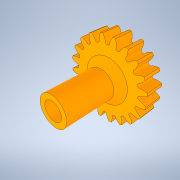
# Autodesk Inventor part: Шестерня мотора
Saved by Autodesk Inventor 2021.1 (Build 251245010, 245A)
## iProperties
Created: 2026-05-06
Part Number: Шестерня мотора
Material: Generic
Document SubType Name: Modeling
Designer: Андрей Тарасов
Density: 1 g/cm^3
Appearance: Default
Author: Андрей Тарасов
Autodesk Inventor part; units mm, degrees
ref_plane "YZ Plane" through (0, 0, 0) normal (1, 0, 0) x (0, 1, 0)
ref_plane "XZ Plane" through (0, 0, 0) normal (0, 1, 0) x (-1, 0, 0)
ref_plane "XY Plane" through (0, 0, 0) normal (0, 0, 1) x (1, 0, 0)
sketch "Sketch1" plane through (0, 0, 0) normal (0, 0, 1) x (1, 0, 0)
  spline S0 degree 3 poles (-1.3768, 10.9135) (-1.3416, 10.8686) (-1.2712, 10.7789) (-1.1713, 10.64) (-1.0757, 10.4981) (-0.9853, 10.3528) (-0.9005, 10.2042) (-0.8221, 10.0521) (-0.7507, 9.8965) (-0.6878, 9.7374) (-0.6438, 9.6016) (-0.616, 9.4911) (-0.5991, 9.407) (-0.5929, 9.3216) (-0.5783, 9.2373) (-0.5604, 9.1536) (-0.5337, 9.0722) (-0.5001, 8.9934) (-0.4629, 8.9323) (-0.4286, 8.8868) (-0.3992, 8.8556) (-0.3672, 8.8271) (-0.3323, 8.8024) (-0.2946, 8.782) (-0.2551, 8.7654) (-0.2137, 8.7543) (-0.1284, 8.7448) (0, 8.7541) (0.1284, 8.7448) (0.2137, 8.7543) (0.2551, 8.7654) (0.2946, 8.782) (0.3323, 8.8024) (0.3672, 8.8271) (0.3992, 8.8556) (0.4286, 8.8868) (0.4629, 8.9323) (0.5001, 8.9934) (0.5337, 9.0722) (0.5604, 9.1536) (0.5783, 9.2373) (0.5929, 9.3216) (0.5991, 9.407) (0.616, 9.4911) (0.6438, 9.6016) (0.6878, 9.7374) (0.7507, 9.8965) (0.8221, 10.0521) (0.9005, 10.2042) (0.9853, 10.3528) (1.0757, 10.4981) (1.1713, 10.64) (1.2712, 10.7789) (1.3416, 10.8686) (1.3768, 10.9135) knots 0 0 0 0 0.017107 0.034214 0.051321 0.068427 0.085534 0.10264 0.119746 0.136852 0.153955 0.162508 0.17106 0.179613 0.188166 0.196719 0.20527 0.213818 0.222364 0.22664 0.230917 0.235193 0.239468 0.24374 0.248014 0.252292 0.256565 0.273669 0.290774 0.295047 0.299325 0.303599 0.307871 0.312146 0.316422 0.320699 0.324975 0.333521 0.342069 0.35062 0.359172 0.367726 0.376279 0.384831 0.393384 0.410487 0.427593 0.444699 0.461805 0.478912 0.496018 0.513125 0.530232 0.547339 0.547339 0.547339 0.547339
  circle A0 centre (0, 0) radius 8.75 construction
  circle A1 centre (0, 0) radius 9.3969 construction
  circle A2 centre (0, 0) radius 10 construction
  circle A3 centre (0, 0) radius 11
  spline S1 degree 3 poles (-4.6819, 9.9539) (-4.6345, 9.9221) (-4.5399, 9.8585) (-4.4019, 9.7573) (-4.2671, 9.6518) (-4.1363, 9.5416) (-4.0097, 9.4264) (-3.8881, 9.3061) (-3.7722, 9.1802) (-3.6632, 9.0483) (-3.5794, 8.9328) (-3.5187, 8.8362) (-3.4768, 8.7615) (-3.4444, 8.6822) (-3.4045, 8.6065) (-3.3616, 8.5324) (-3.311, 8.4633) (-3.2548, 8.3987) (-3.2005, 8.3521) (-3.1538, 8.3194) (-3.1162, 8.2988) (-3.077, 8.2816) (-3.0361, 8.2689) (-2.994, 8.2612) (-2.9513, 8.2575) (-2.9084, 8.2598) (-2.8244, 8.2771) (-2.7052, 8.3257) (-2.5801, 8.3565) (-2.502, 8.3918) (-2.466, 8.4152) (-2.4336, 8.4432) (-2.4041, 8.4742) (-2.3785, 8.5086) (-2.3568, 8.5455) (-2.3385, 8.5843) (-2.32, 8.6382) (-2.3034, 8.7078) (-2.2959, 8.7931) (-2.2957, 8.8787) (-2.3045, 8.9639) (-2.3166, 9.0486) (-2.3371, 9.1318) (-2.3471, 9.2169) (-2.3548, 9.3306) (-2.3549, 9.4734) (-2.3442, 9.6442) (-2.3244, 9.8141) (-2.2968, 9.983) (-2.2621, 10.1506) (-2.221, 10.3167) (-2.1739, 10.4812) (-2.1218, 10.6441) (-2.0826, 10.7513) (-2.063, 10.8048) knots 0 0 0 0 0.017107 0.034214 0.051321 0.068427 0.085534 0.10264 0.119746 0.136852 0.153955 0.162508 0.17106 0.179613 0.188166 0.196719 0.20527 0.213818 0.222364 0.22664 0.230917 0.235193 0.239468 0.24374 0.248014 0.252292 0.256565 0.273669 0.290774 0.295047 0.299325 0.303599 0.307871 0.312146 0.316422 0.320699 0.324975 0.333521 0.342069 0.35062 0.359172 0.367726 0.376279 0.384831 0.393384 0.410487 0.427593 0.444699 0.461805 0.478912 0.496018 0.513125 0.530232 0.547339 0.547339 0.547339 0.547339
  spline S2 degree 3 poles (-7.5287, 8.0199) (-7.4738, 8.0043) (-7.3641, 7.9731) (-7.2016, 7.9194) (-7.0409, 7.8608) (-6.8824, 7.7964) (-6.7264, 7.726) (-6.5735, 7.6491) (-6.4244, 7.5652) (-6.28, 7.4734) (-6.1646, 7.3895) (-6.077, 7.3164) (-6.014, 7.2583) (-5.9588, 7.1928) (-5.8974, 7.1332) (-5.8337, 7.076) (-5.7643, 7.0259) (-5.6908, 6.9818) (-5.6248, 6.9543) (-5.5703, 6.9376) (-5.5282, 6.9296) (-5.4855, 6.9254) (-5.4427, 6.926) (-5.4003, 6.9316) (-5.3585, 6.9414) (-5.3185, 6.9568) (-5.244, 6.9992) (-5.1456, 7.0823) (-5.0362, 7.1502) (-4.9728, 7.2079) (-4.9458, 7.2413) (-4.9236, 7.2779) (-4.9051, 7.3166) (-4.8913, 7.3571) (-4.8822, 7.399) (-4.8768, 7.4415) (-4.8758, 7.4985) (-4.8815, 7.5698) (-4.9008, 7.6533) (-4.927, 7.7348) (-4.9617, 7.813) (-4.9994, 7.8899) (-5.0446, 7.9626) (-5.0804, 8.0405) (-5.1228, 8.1463) (-5.167, 8.282) (-5.2097, 8.4477) (-5.2434, 8.6155) (-5.2693, 8.7847) (-5.2881, 8.9547) (-5.3003, 9.1254) (-5.3064, 9.2964) (-5.3072, 9.4675) (-5.303, 9.5815) (-5.3009, 9.6385) knots 0 0 0 0 0.017107 0.034214 0.051321 0.068427 0.085534 0.10264 0.119746 0.136852 0.153955 0.162508 0.17106 0.179613 0.188166 0.196719 0.20527 0.213818 0.222364 0.22664 0.230917 0.235193 0.239468 0.24374 0.248014 0.252292 0.256565 0.273669 0.290774 0.295047 0.299325 0.303599 0.307871 0.312146 0.316422 0.320699 0.324975 0.333521 0.342069 0.35062 0.359172 0.367726 0.376279 0.384831 0.393384 0.410487 0.427593 0.444699 0.461805 0.478912 0.496018 0.513125 0.530232 0.547339 0.547339 0.547339 0.547339
  spline S3 degree 3 poles (-9.6385, 5.3009) (-9.5815, 5.303) (-9.4675, 5.3072) (-9.2964, 5.3064) (-9.1254, 5.3003) (-8.9547, 5.2881) (-8.7847, 5.2693) (-8.6155, 5.2434) (-8.4477, 5.2097) (-8.282, 5.167) (-8.1463, 5.1228) (-8.0405, 5.0804) (-7.9626, 5.0446) (-7.8899, 4.9994) (-7.813, 4.9617) (-7.7348, 4.927) (-7.6533, 4.9008) (-7.5698, 4.8815) (-7.4985, 4.8758) (-7.4415, 4.8768) (-7.399, 4.8822) (-7.3571, 4.8913) (-7.3166, 4.9051) (-7.2779, 4.9236) (-7.2413, 4.9458) (-7.2079, 4.9728) (-7.1502, 5.0362) (-7.0823, 5.1456) (-6.9992, 5.244) (-6.9568, 5.3185) (-6.9414, 5.3585) (-6.9316, 5.4003) (-6.926, 5.4427) (-6.9254, 5.4855) (-6.9296, 5.5282) (-6.9376, 5.5703) (-6.9543, 5.6248) (-6.9818, 5.6908) (-7.0259, 5.7643) (-7.076, 5.8337) (-7.1332, 5.8974) (-7.1928, 5.9588) (-7.2583, 6.014) (-7.3164, 6.077) (-7.3895, 6.1646) (-7.4734, 6.28) (-7.5652, 6.4244) (-7.6491, 6.5735) (-7.726, 6.7264) (-7.7964, 6.8824) (-7.8608, 7.0409) (-7.9194, 7.2016) (-7.9731, 7.3641) (-8.0043, 7.4738) (-8.0199, 7.5287) knots 0 0 0 0 0.017107 0.034214 0.051321 0.068427 0.085534 0.10264 0.119746 0.136852 0.153955 0.162508 0.17106 0.179613 0.188166 0.196719 0.20527 0.213818 0.222364 0.22664 0.230917 0.235193 0.239468 0.24374 0.248014 0.252292 0.256565 0.273669 0.290774 0.295047 0.299325 0.303599 0.307871 0.312146 0.316422 0.320699 0.324975 0.333521 0.342069 0.35062 0.359172 0.367726 0.376279 0.384831 0.393384 0.410487 0.427593 0.444699 0.461805 0.478912 0.496018 0.513125 0.530232 0.547339 0.547339 0.547339 0.547339
  spline S4 degree 3 poles (-10.8048, 2.063) (-10.7513, 2.0826) (-10.6441, 2.1218) (-10.4812, 2.1739) (-10.3167, 2.221) (-10.1506, 2.2621) (-9.983, 2.2968) (-9.8141, 2.3244) (-9.6442, 2.3442) (-9.4734, 2.3549) (-9.3306, 2.3548) (-9.2169, 2.3471) (-9.1318, 2.3371) (-9.0486, 2.3166) (-8.9639, 2.3045) (-8.8787, 2.2957) (-8.7931, 2.2959) (-8.7078, 2.3034) (-8.6382, 2.32) (-8.5843, 2.3385) (-8.5455, 2.3568) (-8.5086, 2.3785) (-8.4742, 2.4041) (-8.4432, 2.4336) (-8.4152, 2.466) (-8.3918, 2.502) (-8.3565, 2.5801) (-8.3257, 2.7052) (-8.2771, 2.8244) (-8.2598, 2.9084) (-8.2575, 2.9513) (-8.2612, 2.994) (-8.2689, 3.0361) (-8.2816, 3.077) (-8.2988, 3.1162) (-8.3194, 3.1538) (-8.3521, 3.2005) (-8.3987, 3.2548) (-8.4633, 3.311) (-8.5324, 3.3616) (-8.6065, 3.4045) (-8.6822, 3.4444) (-8.7615, 3.4768) (-8.8362, 3.5187) (-8.9328, 3.5794) (-9.0483, 3.6632) (-9.1802, 3.7722) (-9.3061, 3.8881) (-9.4264, 4.0097) (-9.5416, 4.1363) (-9.6518, 4.2671) (-9.7573, 4.4019) (-9.8585, 4.5399) (-9.9221, 4.6345) (-9.9539, 4.6819) knots 0 0 0 0 0.017107 0.034214 0.051321 0.068427 0.085534 0.10264 0.119746 0.136852 0.153955 0.162508 0.17106 0.179613 0.188166 0.196719 0.20527 0.213818 0.222364 0.22664 0.230917 0.235193 0.239468 0.24374 0.248014 0.252292 0.256565 0.273669 0.290774 0.295047 0.299325 0.303599 0.307871 0.312146 0.316422 0.320699 0.324975 0.333521 0.342069 0.35062 0.359172 0.367726 0.376279 0.384831 0.393384 0.410487 0.427593 0.444699 0.461805 0.478912 0.496018 0.513125 0.530232 0.547339 0.547339 0.547339 0.547339
  spline S5 degree 3 poles (-10.9135, -1.3768) (-10.8686, -1.3416) (-10.7789, -1.2712) (-10.64, -1.1713) (-10.4981, -1.0757) (-10.3528, -0.9853) (-10.2042, -0.9005) (-10.0521, -0.8221) (-9.8965, -0.7507) (-9.7374, -0.6878) (-9.6016, -0.6438) (-9.4911, -0.616) (-9.407, -0.5991) (-9.3216, -0.5929) (-9.2373, -0.5783) (-9.1536, -0.5604) (-9.0722, -0.5337) (-8.9934, -0.5001) (-8.9323, -0.4629) (-8.8868, -0.4286) (-8.8556, -0.3992) (-8.8271, -0.3672) (-8.8024, -0.3323) (-8.782, -0.2946) (-8.7654, -0.2551) (-8.7543, -0.2137) (-8.7448, -0.1284) (-8.7541, 0) (-8.7448, 0.1284) (-8.7543, 0.2137) (-8.7654, 0.2551) (-8.782, 0.2946) (-8.8024, 0.3323) (-8.8271, 0.3672) (-8.8556, 0.3992) (-8.8868, 0.4286) (-8.9323, 0.4629) (-8.9934, 0.5001) (-9.0722, 0.5337) (-9.1536, 0.5604) (-9.2373, 0.5783) (-9.3216, 0.5929) (-9.407, 0.5991) (-9.4911, 0.616) (-9.6016, 0.6438) (-9.7374, 0.6878) (-9.8965, 0.7507) (-10.0521, 0.8221) (-10.2042, 0.9005) (-10.3528, 0.9853) (-10.4981, 1.0757) (-10.64, 1.1713) (-10.7789, 1.2712) (-10.8686, 1.3416) (-10.9135, 1.3768) knots 0 0 0 0 0.017107 0.034214 0.051321 0.068427 0.085534 0.10264 0.119746 0.136852 0.153955 0.162508 0.17106 0.179613 0.188166 0.196719 0.20527 0.213818 0.222364 0.22664 0.230917 0.235193 0.239468 0.24374 0.248014 0.252292 0.256565 0.273669 0.290774 0.295047 0.299325 0.303599 0.307871 0.312146 0.316422 0.320699 0.324975 0.333521 0.342069 0.35062 0.359172 0.367726 0.376279 0.384831 0.393384 0.410487 0.427593 0.444699 0.461805 0.478912 0.496018 0.513125 0.530232 0.547339 0.547339 0.547339 0.547339
  spline S6 degree 3 poles (-9.9539, -4.6819) (-9.9221, -4.6345) (-9.8585, -4.5399) (-9.7573, -4.4019) (-9.6518, -4.2671) (-9.5416, -4.1363) (-9.4264, -4.0097) (-9.3061, -3.8881) (-9.1802, -3.7722) (-9.0483, -3.6632) (-8.9328, -3.5794) (-8.8362, -3.5187) (-8.7615, -3.4768) (-8.6822, -3.4444) (-8.6065, -3.4045) (-8.5324, -3.3616) (-8.4633, -3.311) (-8.3987, -3.2548) (-8.3521, -3.2005) (-8.3194, -3.1538) (-8.2988, -3.1162) (-8.2816, -3.077) (-8.2689, -3.0361) (-8.2612, -2.994) (-8.2575, -2.9513) (-8.2598, -2.9084) (-8.2771, -2.8244) (-8.3257, -2.7052) (-8.3565, -2.5801) (-8.3918, -2.502) (-8.4152, -2.466) (-8.4432, -2.4336) (-8.4742, -2.4041) (-8.5086, -2.3785) (-8.5455, -2.3568) (-8.5843, -2.3385) (-8.6382, -2.32) (-8.7078, -2.3034) (-8.7931, -2.2959) (-8.8787, -2.2957) (-8.9639, -2.3045) (-9.0486, -2.3166) (-9.1318, -2.3371) (-9.2169, -2.3471) (-9.3306, -2.3548) (-9.4734, -2.3549) (-9.6442, -2.3442) (-9.8141, -2.3244) (-9.983, -2.2968) (-10.1506, -2.2621) (-10.3167, -2.221) (-10.4812, -2.1739) (-10.6441, -2.1218) (-10.7513, -2.0826) (-10.8048, -2.063) knots 0 0 0 0 0.017107 0.034214 0.051321 0.068427 0.085534 0.10264 0.119746 0.136852 0.153955 0.162508 0.17106 0.179613 0.188166 0.196719 0.20527 0.213818 0.222364 0.22664 0.230917 0.235193 0.239468 0.24374 0.248014 0.252292 0.256565 0.273669 0.290774 0.295047 0.299325 0.303599 0.307871 0.312146 0.316422 0.320699 0.324975 0.333521 0.342069 0.35062 0.359172 0.367726 0.376279 0.384831 0.393384 0.410487 0.427593 0.444699 0.461805 0.478912 0.496018 0.513125 0.530232 0.547339 0.547339 0.547339 0.547339
  spline S7 degree 3 poles (-8.0199, -7.5287) (-8.0043, -7.4738) (-7.9731, -7.3641) (-7.9194, -7.2016) (-7.8608, -7.0409) (-7.7964, -6.8824) (-7.726, -6.7264) (-7.6491, -6.5735) (-7.5652, -6.4244) (-7.4734, -6.28) (-7.3895, -6.1646) (-7.3164, -6.077) (-7.2583, -6.014) (-7.1928, -5.9588) (-7.1332, -5.8974) (-7.076, -5.8337) (-7.0259, -5.7643) (-6.9818, -5.6908) (-6.9543, -5.6248) (-6.9376, -5.5703) (-6.9296, -5.5282) (-6.9254, -5.4855) (-6.926, -5.4427) (-6.9316, -5.4003) (-6.9414, -5.3585) (-6.9568, -5.3185) (-6.9992, -5.244) (-7.0823, -5.1456) (-7.1502, -5.0362) (-7.2079, -4.9728) (-7.2413, -4.9458) (-7.2779, -4.9236) (-7.3166, -4.9051) (-7.3571, -4.8913) (-7.399, -4.8822) (-7.4415, -4.8768) (-7.4985, -4.8758) (-7.5698, -4.8815) (-7.6533, -4.9008) (-7.7348, -4.927) (-7.813, -4.9617) (-7.8899, -4.9994) (-7.9626, -5.0446) (-8.0405, -5.0804) (-8.1463, -5.1228) (-8.282, -5.167) (-8.4477, -5.2097) (-8.6155, -5.2434) (-8.7847, -5.2693) (-8.9547, -5.2881) (-9.1254, -5.3003) (-9.2964, -5.3064) (-9.4675, -5.3072) (-9.5815, -5.303) (-9.6385, -5.3009) knots 0 0 0 0 0.017107 0.034214 0.051321 0.068427 0.085534 0.10264 0.119746 0.136852 0.153955 0.162508 0.17106 0.179613 0.188166 0.196719 0.20527 0.213818 0.222364 0.22664 0.230917 0.235193 0.239468 0.24374 0.248014 0.252292 0.256565 0.273669 0.290774 0.295047 0.299325 0.303599 0.307871 0.312146 0.316422 0.320699 0.324975 0.333521 0.342069 0.35062 0.359172 0.367726 0.376279 0.384831 0.393384 0.410487 0.427593 0.444699 0.461805 0.478912 0.496018 0.513125 0.530232 0.547339 0.547339 0.547339 0.547339
  spline S8 degree 3 poles (-5.3009, -9.6385) (-5.303, -9.5815) (-5.3072, -9.4675) (-5.3064, -9.2964) (-5.3003, -9.1254) (-5.2881, -8.9547) (-5.2693, -8.7847) (-5.2434, -8.6155) (-5.2097, -8.4477) (-5.167, -8.282) (-5.1228, -8.1463) (-5.0804, -8.0405) (-5.0446, -7.9626) (-4.9994, -7.8899) (-4.9617, -7.813) (-4.927, -7.7348) (-4.9008, -7.6533) (-4.8815, -7.5698) (-4.8758, -7.4985) (-4.8768, -7.4415) (-4.8822, -7.399) (-4.8913, -7.3571) (-4.9051, -7.3166) (-4.9236, -7.2779) (-4.9458, -7.2413) (-4.9728, -7.2079) (-5.0362, -7.1502) (-5.1456, -7.0823) (-5.244, -6.9992) (-5.3185, -6.9568) (-5.3585, -6.9414) (-5.4003, -6.9316) (-5.4427, -6.926) (-5.4855, -6.9254) (-5.5282, -6.9296) (-5.5703, -6.9376) (-5.6248, -6.9543) (-5.6908, -6.9818) (-5.7643, -7.0259) (-5.8337, -7.076) (-5.8974, -7.1332) (-5.9588, -7.1928) (-6.014, -7.2583) (-6.077, -7.3164) (-6.1646, -7.3895) (-6.28, -7.4734) (-6.4244, -7.5652) (-6.5735, -7.6491) (-6.7264, -7.726) (-6.8824, -7.7964) (-7.0409, -7.8608) (-7.2016, -7.9194) (-7.3641, -7.9731) (-7.4738, -8.0043) (-7.5287, -8.0199) knots 0 0 0 0 0.017107 0.034214 0.051321 0.068427 0.085534 0.10264 0.119746 0.136852 0.153955 0.162508 0.17106 0.179613 0.188166 0.196719 0.20527 0.213818 0.222364 0.22664 0.230917 0.235193 0.239468 0.24374 0.248014 0.252292 0.256565 0.273669 0.290774 0.295047 0.299325 0.303599 0.307871 0.312146 0.316422 0.320699 0.324975 0.333521 0.342069 0.35062 0.359172 0.367726 0.376279 0.384831 0.393384 0.410487 0.427593 0.444699 0.461805 0.478912 0.496018 0.513125 0.530232 0.547339 0.547339 0.547339 0.547339
  spline S9 degree 3 poles (-2.063, -10.8048) (-2.0826, -10.7513) (-2.1218, -10.6441) (-2.1739, -10.4812) (-2.221, -10.3167) (-2.2621, -10.1506) (-2.2968, -9.983) (-2.3244, -9.8141) (-2.3442, -9.6442) (-2.3549, -9.4734) (-2.3548, -9.3306) (-2.3471, -9.2169) (-2.3371, -9.1318) (-2.3166, -9.0486) (-2.3045, -8.9639) (-2.2957, -8.8787) (-2.2959, -8.7931) (-2.3034, -8.7078) (-2.32, -8.6382) (-2.3385, -8.5843) (-2.3568, -8.5455) (-2.3785, -8.5086) (-2.4041, -8.4742) (-2.4336, -8.4432) (-2.466, -8.4152) (-2.502, -8.3918) (-2.5801, -8.3565) (-2.7052, -8.3257) (-2.8244, -8.2771) (-2.9084, -8.2598) (-2.9513, -8.2575) (-2.994, -8.2612) (-3.0361, -8.2689) (-3.077, -8.2816) (-3.1162, -8.2988) (-3.1538, -8.3194) (-3.2005, -8.3521) (-3.2548, -8.3987) (-3.311, -8.4633) (-3.3616, -8.5324) (-3.4045, -8.6065) (-3.4444, -8.6822) (-3.4768, -8.7615) (-3.5187, -8.8362) (-3.5794, -8.9328) (-3.6632, -9.0483) (-3.7722, -9.1802) (-3.8881, -9.3061) (-4.0097, -9.4264) (-4.1363, -9.5416) (-4.2671, -9.6518) (-4.4019, -9.7573) (-4.5399, -9.8585) (-4.6345, -9.9221) (-4.6819, -9.9539) knots 0 0 0 0 0.017107 0.034214 0.051321 0.068427 0.085534 0.10264 0.119746 0.136852 0.153955 0.162508 0.17106 0.179613 0.188166 0.196719 0.20527 0.213818 0.222364 0.22664 0.230917 0.235193 0.239468 0.24374 0.248014 0.252292 0.256565 0.273669 0.290774 0.295047 0.299325 0.303599 0.307871 0.312146 0.316422 0.320699 0.324975 0.333521 0.342069 0.35062 0.359172 0.367726 0.376279 0.384831 0.393384 0.410487 0.427593 0.444699 0.461805 0.478912 0.496018 0.513125 0.530232 0.547339 0.547339 0.547339 0.547339
  spline S10 degree 3 poles (1.3768, -10.9135) (1.3416, -10.8686) (1.2712, -10.7789) (1.1713, -10.64) (1.0757, -10.4981) (0.9853, -10.3528) (0.9005, -10.2042) (0.8221, -10.0521) (0.7507, -9.8965) (0.6878, -9.7374) (0.6438, -9.6016) (0.616, -9.4911) (0.5991, -9.407) (0.5929, -9.3216) (0.5783, -9.2373) (0.5604, -9.1536) (0.5337, -9.0722) (0.5001, -8.9934) (0.4629, -8.9323) (0.4286, -8.8868) (0.3992, -8.8556) (0.3672, -8.8271) (0.3323, -8.8024) (0.2946, -8.782) (0.2551, -8.7654) (0.2137, -8.7543) (0.1284, -8.7448) (0, -8.7541) (-0.1284, -8.7448) (-0.2137, -8.7543) (-0.2551, -8.7654) (-0.2946, -8.782) (-0.3323, -8.8024) (-0.3672, -8.8271) (-0.3992, -8.8556) (-0.4286, -8.8868) (-0.4629, -8.9323) (-0.5001, -8.9934) (-0.5337, -9.0722) (-0.5604, -9.1536) (-0.5783, -9.2373) (-0.5929, -9.3216) (-0.5991, -9.407) (-0.616, -9.4911) (-0.6438, -9.6016) (-0.6878, -9.7374) (-0.7507, -9.8965) (-0.8221, -10.0521) (-0.9005, -10.2042) (-0.9853, -10.3528) (-1.0757, -10.4981) (-1.1713, -10.64) (-1.2712, -10.7789) (-1.3416, -10.8686) (-1.3768, -10.9135) knots 0 0 0 0 0.017107 0.034214 0.051321 0.068427 0.085534 0.10264 0.119746 0.136852 0.153955 0.162508 0.17106 0.179613 0.188166 0.196719 0.20527 0.213818 0.222364 0.22664 0.230917 0.235193 0.239468 0.24374 0.248014 0.252292 0.256565 0.273669 0.290774 0.295047 0.299325 0.303599 0.307871 0.312146 0.316422 0.320699 0.324975 0.333521 0.342069 0.35062 0.359172 0.367726 0.376279 0.384831 0.393384 0.410487 0.427593 0.444699 0.461805 0.478912 0.496018 0.513125 0.530232 0.547339 0.547339 0.547339 0.547339
  spline S11 degree 3 poles (4.6819, -9.9539) (4.6345, -9.9221) (4.5399, -9.8585) (4.4019, -9.7573) (4.2671, -9.6518) (4.1363, -9.5416) (4.0097, -9.4264) (3.8881, -9.3061) (3.7722, -9.1802) (3.6632, -9.0483) (3.5794, -8.9328) (3.5187, -8.8362) (3.4768, -8.7615) (3.4444, -8.6822) (3.4045, -8.6065) (3.3616, -8.5324) (3.311, -8.4633) (3.2548, -8.3987) (3.2005, -8.3521) (3.1538, -8.3194) (3.1162, -8.2988) (3.077, -8.2816) (3.0361, -8.2689) (2.994, -8.2612) (2.9513, -8.2575) (2.9084, -8.2598) (2.8244, -8.2771) (2.7052, -8.3257) (2.5801, -8.3565) (2.502, -8.3918) (2.466, -8.4152) (2.4336, -8.4432) (2.4041, -8.4742) (2.3785, -8.5086) (2.3568, -8.5455) (2.3385, -8.5843) (2.32, -8.6382) (2.3034, -8.7078) (2.2959, -8.7931) (2.2957, -8.8787) (2.3045, -8.9639) (2.3166, -9.0486) (2.3371, -9.1318) (2.3471, -9.2169) (2.3548, -9.3306) (2.3549, -9.4734) (2.3442, -9.6442) (2.3244, -9.8141) (2.2968, -9.983) (2.2621, -10.1506) (2.221, -10.3167) (2.1739, -10.4812) (2.1218, -10.6441) (2.0826, -10.7513) (2.063, -10.8048) knots 0 0 0 0 0.017107 0.034214 0.051321 0.068427 0.085534 0.10264 0.119746 0.136852 0.153955 0.162508 0.17106 0.179613 0.188166 0.196719 0.20527 0.213818 0.222364 0.22664 0.230917 0.235193 0.239468 0.24374 0.248014 0.252292 0.256565 0.273669 0.290774 0.295047 0.299325 0.303599 0.307871 0.312146 0.316422 0.320699 0.324975 0.333521 0.342069 0.35062 0.359172 0.367726 0.376279 0.384831 0.393384 0.410487 0.427593 0.444699 0.461805 0.478912 0.496018 0.513125 0.530232 0.547339 0.547339 0.547339 0.547339
  spline S12 degree 3 poles (7.5287, -8.0199) (7.4738, -8.0043) (7.3641, -7.9731) (7.2016, -7.9194) (7.0409, -7.8608) (6.8824, -7.7964) (6.7264, -7.726) (6.5735, -7.6491) (6.4244, -7.5652) (6.28, -7.4734) (6.1646, -7.3895) (6.077, -7.3164) (6.014, -7.2583) (5.9588, -7.1928) (5.8974, -7.1332) (5.8337, -7.076) (5.7643, -7.0259) (5.6908, -6.9818) (5.6248, -6.9543) (5.5703, -6.9376) (5.5282, -6.9296) (5.4855, -6.9254) (5.4427, -6.926) (5.4003, -6.9316) (5.3585, -6.9414) (5.3185, -6.9568) (5.244, -6.9992) (5.1456, -7.0823) (5.0362, -7.1502) (4.9728, -7.2079) (4.9458, -7.2413) (4.9236, -7.2779) (4.9051, -7.3166) (4.8913, -7.3571) (4.8822, -7.399) (4.8768, -7.4415) (4.8758, -7.4985) (4.8815, -7.5698) (4.9008, -7.6533) (4.927, -7.7348) (4.9617, -7.813) (4.9994, -7.8899) (5.0446, -7.9626) (5.0804, -8.0405) (5.1228, -8.1463) (5.167, -8.282) (5.2097, -8.4477) (5.2434, -8.6155) (5.2693, -8.7847) (5.2881, -8.9547) (5.3003, -9.1254) (5.3064, -9.2964) (5.3072, -9.4675) (5.303, -9.5815) (5.3009, -9.6385) knots 0 0 0 0 0.017107 0.034214 0.051321 0.068427 0.085534 0.10264 0.119746 0.136852 0.153955 0.162508 0.17106 0.179613 0.188166 0.196719 0.20527 0.213818 0.222364 0.22664 0.230917 0.235193 0.239468 0.24374 0.248014 0.252292 0.256565 0.273669 0.290774 0.295047 0.299325 0.303599 0.307871 0.312146 0.316422 0.320699 0.324975 0.333521 0.342069 0.35062 0.359172 0.367726 0.376279 0.384831 0.393384 0.410487 0.427593 0.444699 0.461805 0.478912 0.496018 0.513125 0.530232 0.547339 0.547339 0.547339 0.547339
  spline S13 degree 3 poles (9.6385, -5.3009) (9.5815, -5.303) (9.4675, -5.3072) (9.2964, -5.3064) (9.1254, -5.3003) (8.9547, -5.2881) (8.7847, -5.2693) (8.6155, -5.2434) (8.4477, -5.2097) (8.282, -5.167) (8.1463, -5.1228) (8.0405, -5.0804) (7.9626, -5.0446) (7.8899, -4.9994) (7.813, -4.9617) (7.7348, -4.927) (7.6533, -4.9008) (7.5698, -4.8815) (7.4985, -4.8758) (7.4415, -4.8768) (7.399, -4.8822) (7.3571, -4.8913) (7.3166, -4.9051) (7.2779, -4.9236) (7.2413, -4.9458) (7.2079, -4.9728) (7.1502, -5.0362) (7.0823, -5.1456) (6.9992, -5.244) (6.9568, -5.3185) (6.9414, -5.3585) (6.9316, -5.4003) (6.926, -5.4427) (6.9254, -5.4855) (6.9296, -5.5282) (6.9376, -5.5703) (6.9543, -5.6248) (6.9818, -5.6908) (7.0259, -5.7643) (7.076, -5.8337) (7.1332, -5.8974) (7.1928, -5.9588) (7.2583, -6.014) (7.3164, -6.077) (7.3895, -6.1646) (7.4734, -6.28) (7.5652, -6.4244) (7.6491, -6.5735) (7.726, -6.7264) (7.7964, -6.8824) (7.8608, -7.0409) (7.9194, -7.2016) (7.9731, -7.3641) (8.0043, -7.4738) (8.0199, -7.5287) knots 0 0 0 0 0.017107 0.034214 0.051321 0.068427 0.085534 0.10264 0.119746 0.136852 0.153955 0.162508 0.17106 0.179613 0.188166 0.196719 0.20527 0.213818 0.222364 0.22664 0.230917 0.235193 0.239468 0.24374 0.248014 0.252292 0.256565 0.273669 0.290774 0.295047 0.299325 0.303599 0.307871 0.312146 0.316422 0.320699 0.324975 0.333521 0.342069 0.35062 0.359172 0.367726 0.376279 0.384831 0.393384 0.410487 0.427593 0.444699 0.461805 0.478912 0.496018 0.513125 0.530232 0.547339 0.547339 0.547339 0.547339
  spline S14 degree 3 poles (10.8048, -2.063) (10.7513, -2.0826) (10.6441, -2.1218) (10.4812, -2.1739) (10.3167, -2.221) (10.1506, -2.2621) (9.983, -2.2968) (9.8141, -2.3244) (9.6442, -2.3442) (9.4734, -2.3549) (9.3306, -2.3548) (9.2169, -2.3471) (9.1318, -2.3371) (9.0486, -2.3166) (8.9639, -2.3045) (8.8787, -2.2957) (8.7931, -2.2959) (8.7078, -2.3034) (8.6382, -2.32) (8.5843, -2.3385) (8.5455, -2.3568) (8.5086, -2.3785) (8.4742, -2.4041) (8.4432, -2.4336) (8.4152, -2.466) (8.3918, -2.502) (8.3565, -2.5801) (8.3257, -2.7052) (8.2771, -2.8244) (8.2598, -2.9084) (8.2575, -2.9513) (8.2612, -2.994) (8.2689, -3.0361) (8.2816, -3.077) (8.2988, -3.1162) (8.3194, -3.1538) (8.3521, -3.2005) (8.3987, -3.2548) (8.4633, -3.311) (8.5324, -3.3616) (8.6065, -3.4045) (8.6822, -3.4444) (8.7615, -3.4768) (8.8362, -3.5187) (8.9328, -3.5794) (9.0483, -3.6632) (9.1802, -3.7722) (9.3061, -3.8881) (9.4264, -4.0097) (9.5416, -4.1363) (9.6518, -4.2671) (9.7573, -4.4019) (9.8585, -4.5399) (9.9221, -4.6345) (9.9539, -4.6819) knots 0 0 0 0 0.017107 0.034214 0.051321 0.068427 0.085534 0.10264 0.119746 0.136852 0.153955 0.162508 0.17106 0.179613 0.188166 0.196719 0.20527 0.213818 0.222364 0.22664 0.230917 0.235193 0.239468 0.24374 0.248014 0.252292 0.256565 0.273669 0.290774 0.295047 0.299325 0.303599 0.307871 0.312146 0.316422 0.320699 0.324975 0.333521 0.342069 0.35062 0.359172 0.367726 0.376279 0.384831 0.393384 0.410487 0.427593 0.444699 0.461805 0.478912 0.496018 0.513125 0.530232 0.547339 0.547339 0.547339 0.547339
  spline S15 degree 3 poles (10.9135, 1.3768) (10.8686, 1.3416) (10.7789, 1.2712) (10.64, 1.1713) (10.4981, 1.0757) (10.3528, 0.9853) (10.2042, 0.9005) (10.0521, 0.8221) (9.8965, 0.7507) (9.7374, 0.6878) (9.6016, 0.6438) (9.4911, 0.616) (9.407, 0.5991) (9.3216, 0.5929) (9.2373, 0.5783) (9.1536, 0.5604) (9.0722, 0.5337) (8.9934, 0.5001) (8.9323, 0.4629) (8.8868, 0.4286) (8.8556, 0.3992) (8.8271, 0.3672) (8.8024, 0.3323) (8.782, 0.2946) (8.7654, 0.2551) (8.7543, 0.2137) (8.7448, 0.1284) (8.7541, 0) (8.7448, -0.1284) (8.7543, -0.2137) (8.7654, -0.2551) (8.782, -0.2946) (8.8024, -0.3323) (8.8271, -0.3672) (8.8556, -0.3992) (8.8868, -0.4286) (8.9323, -0.4629) (8.9934, -0.5001) (9.0722, -0.5337) (9.1536, -0.5604) (9.2373, -0.5783) (9.3216, -0.5929) (9.407, -0.5991) (9.4911, -0.616) (9.6016, -0.6438) (9.7374, -0.6878) (9.8965, -0.7507) (10.0521, -0.8221) (10.2042, -0.9005) (10.3528, -0.9853) (10.4981, -1.0757) (10.64, -1.1713) (10.7789, -1.2712) (10.8686, -1.3416) (10.9135, -1.3768) knots 0 0 0 0 0.017107 0.034214 0.051321 0.068427 0.085534 0.10264 0.119746 0.136852 0.153955 0.162508 0.17106 0.179613 0.188166 0.196719 0.20527 0.213818 0.222364 0.22664 0.230917 0.235193 0.239468 0.24374 0.248014 0.252292 0.256565 0.273669 0.290774 0.295047 0.299325 0.303599 0.307871 0.312146 0.316422 0.320699 0.324975 0.333521 0.342069 0.35062 0.359172 0.367726 0.376279 0.384831 0.393384 0.410487 0.427593 0.444699 0.461805 0.478912 0.496018 0.513125 0.530232 0.547339 0.547339 0.547339 0.547339
  spline S16 degree 3 poles (9.9539, 4.6819) (9.9221, 4.6345) (9.8585, 4.5399) (9.7573, 4.4019) (9.6518, 4.2671) (9.5416, 4.1363) (9.4264, 4.0097) (9.3061, 3.8881) (9.1802, 3.7722) (9.0483, 3.6632) (8.9328, 3.5794) (8.8362, 3.5187) (8.7615, 3.4768) (8.6822, 3.4444) (8.6065, 3.4045) (8.5324, 3.3616) (8.4633, 3.311) (8.3987, 3.2548) (8.3521, 3.2005) (8.3194, 3.1538) (8.2988, 3.1162) (8.2816, 3.077) (8.2689, 3.0361) (8.2612, 2.994) (8.2575, 2.9513) (8.2598, 2.9084) (8.2771, 2.8244) (8.3257, 2.7052) (8.3565, 2.5801) (8.3918, 2.502) (8.4152, 2.466) (8.4432, 2.4336) (8.4742, 2.4041) (8.5086, 2.3785) (8.5455, 2.3568) (8.5843, 2.3385) (8.6382, 2.32) (8.7078, 2.3034) (8.7931, 2.2959) (8.8787, 2.2957) (8.9639, 2.3045) (9.0486, 2.3166) (9.1318, 2.3371) (9.2169, 2.3471) (9.3306, 2.3548) (9.4734, 2.3549) (9.6442, 2.3442) (9.8141, 2.3244) (9.983, 2.2968) (10.1506, 2.2621) (10.3167, 2.221) (10.4812, 2.1739) (10.6441, 2.1218) (10.7513, 2.0826) (10.8048, 2.063) knots 0 0 0 0 0.017107 0.034214 0.051321 0.068427 0.085534 0.10264 0.119746 0.136852 0.153955 0.162508 0.17106 0.179613 0.188166 0.196719 0.20527 0.213818 0.222364 0.22664 0.230917 0.235193 0.239468 0.24374 0.248014 0.252292 0.256565 0.273669 0.290774 0.295047 0.299325 0.303599 0.307871 0.312146 0.316422 0.320699 0.324975 0.333521 0.342069 0.35062 0.359172 0.367726 0.376279 0.384831 0.393384 0.410487 0.427593 0.444699 0.461805 0.478912 0.496018 0.513125 0.530232 0.547339 0.547339 0.547339 0.547339
  spline S17 degree 3 poles (8.0199, 7.5287) (8.0043, 7.4738) (7.9731, 7.3641) (7.9194, 7.2016) (7.8608, 7.0409) (7.7964, 6.8824) (7.726, 6.7264) (7.6491, 6.5735) (7.5652, 6.4244) (7.4734, 6.28) (7.3895, 6.1646) (7.3164, 6.077) (7.2583, 6.014) (7.1928, 5.9588) (7.1332, 5.8974) (7.076, 5.8337) (7.0259, 5.7643) (6.9818, 5.6908) (6.9543, 5.6248) (6.9376, 5.5703) (6.9296, 5.5282) (6.9254, 5.4855) (6.926, 5.4427) (6.9316, 5.4003) (6.9414, 5.3585) (6.9568, 5.3185) (6.9992, 5.244) (7.0823, 5.1456) (7.1502, 5.0362) (7.2079, 4.9728) (7.2413, 4.9458) (7.2779, 4.9236) (7.3166, 4.9051) (7.3571, 4.8913) (7.399, 4.8822) (7.4415, 4.8768) (7.4985, 4.8758) (7.5698, 4.8815) (7.6533, 4.9008) (7.7348, 4.927) (7.813, 4.9617) (7.8899, 4.9994) (7.9626, 5.0446) (8.0405, 5.0804) (8.1463, 5.1228) (8.282, 5.167) (8.4477, 5.2097) (8.6155, 5.2434) (8.7847, 5.2693) (8.9547, 5.2881) (9.1254, 5.3003) (9.2964, 5.3064) (9.4675, 5.3072) (9.5815, 5.303) (9.6385, 5.3009) knots 0 0 0 0 0.017107 0.034214 0.051321 0.068427 0.085534 0.10264 0.119746 0.136852 0.153955 0.162508 0.17106 0.179613 0.188166 0.196719 0.20527 0.213818 0.222364 0.22664 0.230917 0.235193 0.239468 0.24374 0.248014 0.252292 0.256565 0.273669 0.290774 0.295047 0.299325 0.303599 0.307871 0.312146 0.316422 0.320699 0.324975 0.333521 0.342069 0.35062 0.359172 0.367726 0.376279 0.384831 0.393384 0.410487 0.427593 0.444699 0.461805 0.478912 0.496018 0.513125 0.530232 0.547339 0.547339 0.547339 0.547339
  spline S18 degree 3 poles (5.3009, 9.6385) (5.303, 9.5815) (5.3072, 9.4675) (5.3064, 9.2964) (5.3003, 9.1254) (5.2881, 8.9547) (5.2693, 8.7847) (5.2434, 8.6155) (5.2097, 8.4477) (5.167, 8.282) (5.1228, 8.1463) (5.0804, 8.0405) (5.0446, 7.9626) (4.9994, 7.8899) (4.9617, 7.813) (4.927, 7.7348) (4.9008, 7.6533) (4.8815, 7.5698) (4.8758, 7.4985) (4.8768, 7.4415) (4.8822, 7.399) (4.8913, 7.3571) (4.9051, 7.3166) (4.9236, 7.2779) (4.9458, 7.2413) (4.9728, 7.2079) (5.0362, 7.1502) (5.1456, 7.0823) (5.244, 6.9992) (5.3185, 6.9568) (5.3585, 6.9414) (5.4003, 6.9316) (5.4427, 6.926) (5.4855, 6.9254) (5.5282, 6.9296) (5.5703, 6.9376) (5.6248, 6.9543) (5.6908, 6.9818) (5.7643, 7.0259) (5.8337, 7.076) (5.8974, 7.1332) (5.9588, 7.1928) (6.014, 7.2583) (6.077, 7.3164) (6.1646, 7.3895) (6.28, 7.4734) (6.4244, 7.5652) (6.5735, 7.6491) (6.7264, 7.726) (6.8824, 7.7964) (7.0409, 7.8608) (7.2016, 7.9194) (7.3641, 7.9731) (7.4738, 8.0043) (7.5287, 8.0199) knots 0 0 0 0 0.017107 0.034214 0.051321 0.068427 0.085534 0.10264 0.119746 0.136852 0.153955 0.162508 0.17106 0.179613 0.188166 0.196719 0.20527 0.213818 0.222364 0.22664 0.230917 0.235193 0.239468 0.24374 0.248014 0.252292 0.256565 0.273669 0.290774 0.295047 0.299325 0.303599 0.307871 0.312146 0.316422 0.320699 0.324975 0.333521 0.342069 0.35062 0.359172 0.367726 0.376279 0.384831 0.393384 0.410487 0.427593 0.444699 0.461805 0.478912 0.496018 0.513125 0.530232 0.547339 0.547339 0.547339 0.547339
  spline S19 degree 3 poles (2.063, 10.8048) (2.0826, 10.7513) (2.1218, 10.6441) (2.1739, 10.4812) (2.221, 10.3167) (2.2621, 10.1506) (2.2968, 9.983) (2.3244, 9.8141) (2.3442, 9.6442) (2.3549, 9.4734) (2.3548, 9.3306) (2.3471, 9.2169) (2.3371, 9.1318) (2.3166, 9.0486) (2.3045, 8.9639) (2.2957, 8.8787) (2.2959, 8.7931) (2.3034, 8.7078) (2.32, 8.6382) (2.3385, 8.5843) (2.3568, 8.5455) (2.3785, 8.5086) (2.4041, 8.4742) (2.4336, 8.4432) (2.466, 8.4152) (2.502, 8.3918) (2.5801, 8.3565) (2.7052, 8.3257) (2.8244, 8.2771) (2.9084, 8.2598) (2.9513, 8.2575) (2.994, 8.2612) (3.0361, 8.2689) (3.077, 8.2816) (3.1162, 8.2988) (3.1538, 8.3194) (3.2005, 8.3521) (3.2548, 8.3987) (3.311, 8.4633) (3.3616, 8.5324) (3.4045, 8.6065) (3.4444, 8.6822) (3.4768, 8.7615) (3.5187, 8.8362) (3.5794, 8.9328) (3.6632, 9.0483) (3.7722, 9.1802) (3.8881, 9.3061) (4.0097, 9.4264) (4.1363, 9.5416) (4.2671, 9.6518) (4.4019, 9.7573) (4.5399, 9.8585) (4.6345, 9.9221) (4.6819, 9.9539) knots 0 0 0 0 0.017107 0.034214 0.051321 0.068427 0.085534 0.10264 0.119746 0.136852 0.153955 0.162508 0.17106 0.179613 0.188166 0.196719 0.20527 0.213818 0.222364 0.22664 0.230917 0.235193 0.239468 0.24374 0.248014 0.252292 0.256565 0.273669 0.290774 0.295047 0.299325 0.303599 0.307871 0.312146 0.316422 0.320699 0.324975 0.333521 0.342069 0.35062 0.359172 0.367726 0.376279 0.384831 0.393384 0.410487 0.427593 0.444699 0.461805 0.478912 0.496018 0.513125 0.530232 0.547339 0.547339 0.547339 0.547339
  circle A4 centre (0, 0) radius 2.5
  line L0 (0, -15.4) -> (0, 15.4) construction
  line L1 (-2, -1.5) -> (-2, 1.5)
  point P0 (-1.2722, 10.7782)
  point P1 (-1.172, 10.6395)
  point P2 (-1.0766, 10.4975)
  point P3 (-0.9863, 10.3522)
  point P4 (-0.9016, 10.2036)
  point P5 (-0.8233, 10.0515)
  point P6 (-0.7521, 9.8959)
  point P7 (-0.6895, 9.7368)
  point P8 (-0.6375, 9.5738)
  point P9 (-0.6166, 9.4909)
  point P10 (-0.6009, 9.4068)
  point P11 (-0.5915, 9.3218)
  point P12 (-0.5778, 9.2374)
  point P13 (-0.5589, 9.154)
  point P14 (-0.5325, 9.0726)
  point P15 (-0.4983, 8.9943)
  point P16 (-0.454, 8.9212)
  point P17 (-0.428, 8.8873)
  point P18 (-0.3988, 8.856)
  point P19 (-0.3667, 8.8277)
  point P20 (-0.3318, 8.8031)
  point P21 (-0.2943, 8.7826)
  point P22 (-0.2548, 8.7663)
  point P23 (-0.2134, 8.7553)
  point P24 (-0.171, 8.7501)
  point P25 (0, 8.75)
  point P26 (0.171, 8.7501)
  point P27 (0.2134, 8.7553)
  point P28 (0.2548, 8.7663)
  point P29 (0.2943, 8.7826)
  point P30 (0.3318, 8.8031)
  point P31 (0.3667, 8.8277)
  point P32 (0.3988, 8.856)
  point P33 (0.428, 8.8873)
  point P34 (0.454, 8.9212)
  point P35 (0.4983, 8.9943)
  point P36 (0.5325, 9.0726)
  point P37 (0.5589, 9.154)
  point P38 (0.5778, 9.2374)
  point P39 (0.5915, 9.3218)
  point P40 (0.6009, 9.4068)
  point P41 (0.6166, 9.4909)
  point P42 (0.6375, 9.5738)
  point P43 (0.6895, 9.7368)
  point P44 (0.7521, 9.8959)
  point P45 (0.8233, 10.0515)
  point P46 (0.9016, 10.2036)
  point P47 (0.9863, 10.3522)
  point P48 (1.0766, 10.4975)
  point P49 (1.172, 10.6395)
  point P50 (1.2722, 10.7782)
  point P51 (-2.5412, 8.3747)
  point P52 (-2.5025, 8.3928)
  point P53 (-2.4666, 8.416)
  point P54 (-2.4341, 8.4437)
  point P55 (-2.4047, 8.4748)
  point P56 (-2.3791, 8.509)
  point P57 (-2.3574, 8.5458)
  point P58 (-2.325, 8.6249)
  point P59 (-2.3055, 8.7081)
  point P60 (-2.2971, 8.7931)
  point P61 (-2.3354, 9.1321)
  point P62 (-2.318, 9.0483)
  point P63 (-2.305, 8.9638)
  point P64 (-2.2972, 8.8787)
  point P65 (-2.3393, 8.5845)
  point P66 (-2.3522, 9.3022)
  point P67 (-2.3531, 9.4733)
  point P68 (-2.3427, 9.644)
  point P69 (-2.3464, 9.2169)
  point P70 (-4.5405, 9.8575)
  point P71 (-4.4024, 9.7566)
  point P72 (-4.2678, 9.651)
  point P73 (-4.137, 9.5408)
  point P74 (-4.0105, 9.4256)
  point P75 (-3.889, 9.3052)
  point P76 (-3.7733, 9.1792)
  point P77 (-3.6646, 9.0471)
  point P78 (-3.5647, 8.9083)
  point P79 (-2.7039, 8.3217)
  point P80 (-3.5193, 8.8358)
  point P81 (-3.4784, 8.7607)
  point P82 (-3.4432, 8.6828)
  point P83 (-3.404, 8.6067)
  point P84 (-3.3603, 8.5332)
  point P85 (-3.3101, 8.464)
  point P86 (-3.2533, 8.4001)
  point P87 (-3.1886, 8.3443)
  point P88 (-3.1534, 8.32)
  point P89 (-3.1159, 8.2993)
  point P90 (-3.0767, 8.2823)
  point P91 (-3.0359, 8.2697)
  point P92 (-2.9939, 8.2618)
  point P93 (-2.9513, 8.2585)
  point P94 (-2.9085, 8.2608)
  point P95 (-2.8666, 8.2689)
  point P96 (-2.3231, 9.814)
  point P97 (-2.2956, 9.9828)
  point P98 (-2.261, 10.1503)
  point P99 (-2.22, 10.3164)
  point P100 (-2.1731, 10.4809)
  point P101 (-2.1207, 10.6438)
  point P102 (-5.0048, 7.1795)
  point P103 (-4.9736, 7.2087)
  point P104 (-4.9466, 7.2418)
  point P105 (-4.9242, 7.2783)
  point P106 (-4.9059, 7.3169)
  point P107 (-4.8921, 7.3573)
  point P108 (-4.8828, 7.3991)
  point P109 (-4.8765, 7.4843)
  point P110 (-4.8836, 7.5694)
  point P111 (-4.9019, 7.6529)
  point P112 (-5.043, 7.9635)
  point P113 (-5.0007, 7.8892)
  point P114 (-4.9622, 7.8128)
  point P115 (-4.9284, 7.7342)
  point P116 (-4.8775, 7.4415)
  point P117 (-5.1116, 8.1201)
  point P118 (-5.1653, 8.2825)
  point P119 (-5.2082, 8.4481)
  point P120 (-5.0797, 8.0407)
  point P121 (-7.3645, 7.9719)
  point P122 (-7.2019, 7.9186)
  point P123 (-7.0413, 7.8599)
  point P124 (-6.8828, 7.7954)
  point P125 (-6.7269, 7.7249)
  point P126 (-6.5742, 7.6479)
  point P127 (-6.4252, 7.5639)
  point P128 (-6.2809, 7.4719)
  point P129 (-6.1431, 7.3707)
  point P130 (-5.1431, 7.0789)
  point P131 (-6.0775, 7.3158)
  point P132 (-6.0153, 7.2571)
  point P133 (-5.9578, 7.1938)
  point P134 (-5.897, 7.1336)
  point P135 (-5.8327, 7.0772)
  point P136 (-5.7636, 7.0269)
  point P137 (-5.6898, 6.9837)
  point P138 (-5.611, 6.9506)
  point P139 (-5.5701, 6.9384)
  point P140 (-5.5281, 6.9303)
  point P141 (-5.4855, 6.9262)
  point P142 (-5.4428, 6.9268)
  point P143 (-5.4004, 6.9323)
  point P144 (-5.3588, 6.9423)
  point P145 (-5.3189, 6.9577)
  point P146 (-5.2815, 6.9784)
  point P147 (-5.2421, 8.6157)
  point P148 (-5.2681, 8.7848)
  point P149 (-5.287, 8.9548)
  point P150 (-5.2993, 9.1255)
  point P151 (-5.3055, 9.2964)
  point P152 (-5.306, 9.4675)
  point P153 (-6.9784, 5.2815)
  point P154 (-6.9577, 5.3189)
  point P155 (-6.9423, 5.3588)
  point P156 (-6.9323, 5.4004)
  point P157 (-6.9268, 5.4428)
  point P158 (-6.9262, 5.4855)
  point P159 (-6.9303, 5.5281)
  point P160 (-6.9506, 5.611)
  point P161 (-6.9837, 5.6898)
  point P162 (-7.0269, 5.7636)
  point P163 (-7.2571, 6.0153)
  point P164 (-7.1938, 5.9578)
  point P165 (-7.1336, 5.897)
  point P166 (-7.0772, 5.8327)
  point P167 (-6.9384, 5.5701)
  point P168 (-7.3707, 6.1431)
  point P169 (-7.4719, 6.2809)
  point P170 (-7.5639, 6.4252)
  point P171 (-7.3158, 6.0775)
  point P172 (-9.4675, 5.306)
  point P173 (-9.2964, 5.3055)
  point P174 (-9.1255, 5.2993)
  point P175 (-8.9548, 5.287)
  point P176 (-8.7848, 5.2681)
  point P177 (-8.6157, 5.2421)
  point P178 (-8.4481, 5.2082)
  point P179 (-8.2825, 5.1653)
  point P180 (-8.1201, 5.1116)
  point P181 (-7.0789, 5.1431)
  point P182 (-8.0407, 5.0797)
  point P183 (-7.9635, 5.043)
  point P184 (-7.8892, 5.0007)
  point P185 (-7.8128, 4.9622)
  point P186 (-7.7342, 4.9284)
  point P187 (-7.6529, 4.9019)
  point P188 (-7.5694, 4.8836)
  point P189 (-7.4843, 4.8765)
  point P190 (-7.4415, 4.8775)
  point P191 (-7.3991, 4.8828)
  point P192 (-7.3573, 4.8921)
  point P193 (-7.3169, 4.9059)
  point P194 (-7.2783, 4.9242)
  point P195 (-7.2418, 4.9466)
  point P196 (-7.2087, 4.9736)
  point P197 (-7.1795, 5.0048)
  point P198 (-7.6479, 6.5742)
  point P199 (-7.7249, 6.7269)
  dimension "d4" = 360
  dimension "d6" = 5
  dimension "d7" = 2
  constraints: 4 centre point, 2 end point, 2 point on circle, 1 coincident, 1 vertical, 2202 other
  measures "d6" diameter of A4
  measures "d7" distance between parallel lines of L0 L1
extrude "Выдавливание1" add sketch "Sketch1" against normal blind 5 contours S0 A3 S19 S18 S17 S16 S15 S14 S13 S12 S11 S10 S9 S8 S7 S6 S5 S4 S3 S2 S1 | L1 A4 picked at (-2.0912, -0.3466)
sketch "Эскиз2" plane through (0, 0, 0) normal (0, 0, 1) x (1, 0, 0)
  arc A0 (-2, -1.5) -> (-2, 1.5) centre (0, 0) ccw projected
  circle A1 centre (0, 0) radius 2.5
  circle A2 centre (0, 0) radius 4
  dimension "d10" = 8
  constraints: 2 centre point, 2 coincident, 1 concentric
  measures "d10" diameter of A2
extrude "Выдавливание2" add sketch "Эскиз2" along normal blind 15
sketch "Эскиз3" plane through (0, 0, 0) normal (0, 0, 1) x (1, 0, 0)
  arc A0 (-2, 1.5) -> (-2, -1.5) centre (0, 0) ccw projected
  line L0 (-2, -1.5) -> (-2, 1.5) projected
extrude "Выдавливание3" add sketch "Эскиз3" along normal blind 6
chamfer "Фаска1" distance 2 angle 45 1 edges at (-4, 0, 0)
chamfer "Фаска2" distance 0.6 angle 45 2 edges at (2.5, 0, -5) (-2, 0, -5)
equation "\"d0\" = Ширина_грани"
equation "\"Модуль\" = 1"
equation "\"Угол_зацепления\" = 20deg"
equation "\"Зазор_профиля_зуба\" = 0.25"
equation "\"Радиус_закругления_зуба\" = 0.2386"
equation "\"Диаметр_головки\" = 22"
equation "\"Диаметр_впадин\" = 17.5"
equation "\"Основной_диаметр\" = 18.79385"
equation "\"Средний_диаметр\" = 20"
equation "\"Ширина_грани\" = 5"
equation "\"Коэффициент_смещения\" = 0"
equation "\"Изменение_высоты_головки_зуба\" = 0"
equation "\"Окружной_шаг\" = 3.14159"
equation "\"Общий_сдвиг_инструмента\" = 0"
equation "\"Внутренний\" = 0"
